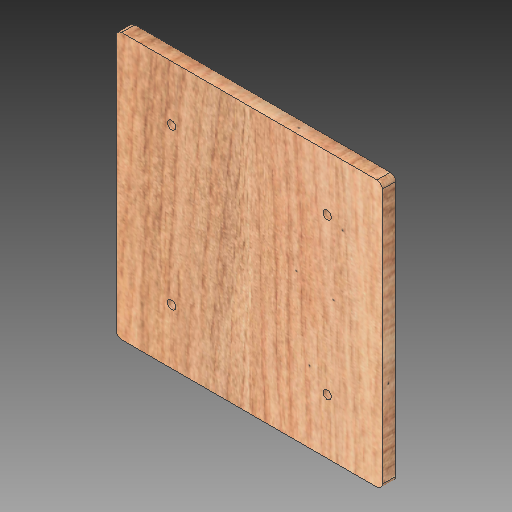
# Autodesk Inventor part: TablaSoporte2
Saved by Autodesk Inventor 2017 (Build 210142000, 142)
## iProperties
Part Number: TablaSoporte2
Material: Madera (abedul)
Document SubType Name: Modeling
Designer: Leonardo
Density: 0.55 g/cm^3
Appearance: Abedul - Natural pulido
Mass: 219.228 g
Surface Area: 884.485 cm^2
Volume: 398.596 cm^3
Author: Leonardo
Autodesk Inventor part; units mm, degrees
ref_plane "YZ Plane" through (0, 0, 0) normal (1, 0, 0) x (0, 1, 0)
ref_plane "XZ Plane" through (0, 0, 0) normal (0, 1, 0) x (-1, 0, 0)
ref_plane "XY Plane" through (0, 0, 0) normal (0, 0, 1) x (1, 0, 0)
ref_plane "Plano de trabajo1" through (0, 0, 150) normal (0, 0, 1) x (1, 0, 0)
sketch "Boceto1" plane through (0, 0, 150) normal (0, 0, 1) x (1, 0, 0)
  line L0 (-96, 100) -> (96, 100)
  line L1 (100, 96) -> (100, -96)
  line L2 (96, -100) -> (-96, -100)
  line L3 (-100, -96) -> (-100, 96)
  line L4 (-100, 100) -> (100, -100) construction
  line L5 (100, 100) -> (-100, -100) construction
  arc A0 (100, 96) -> (96, 100) centre (96, 96) ccw
  arc A1 (-96, 100) -> (-100, 96) centre (-96, 96) ccw
  arc A2 (-100, -96) -> (-96, -100) centre (-96, -96) ccw
  arc A3 (96, -100) -> (100, -96) centre (96, -96) ccw
  circle A4 centre (58.5, 58.5) radius 3.175 projected
  circle A5 centre (-58.5, 58.5) radius 3.175 projected
  circle A6 centre (-58.5, -58.5) radius 3.175 projected
  circle A7 centre (58.5, -58.5) radius 3.175 projected
  point P0 (0, 0)
  dimension "d0" = 200
  dimension "d1" = 200
  dimension "d2" = 4
  constraints: 12 end point, 8 point on circle, 8 point on line, 8 tangent, 4 centre point, 3 equal radius, 2 midpoint, 2 parallel, 1 horizontal, 1 perpendicular
  measures "d0" distance of L4.end L5.end
  measures "d1" distance of L5.start L4.end
  measures "d2" radius of A0
extrude "Extrusión1" add sketch "Boceto1" along normal blind 10
